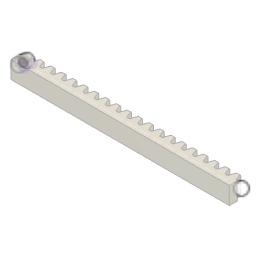
Parametric Rack (Autodesk Fusion 360 design; units mm, degrees)
Autodesk Fusion 360 part; units mm, degrees
sketch "Diameters" plane through (0, 0, 0) normal (0, 1, 0) x (1, 0, 0) in component "Rack"
  line L0 (0, 0) -> (62.8319, 0)
  line L1 (62.8319, 0) -> (62.8319, -4.5)
  line L2 (62.8319, -4.5) -> (0, -4.5)
  line L3 (0, -4.5) -> (0, 0)
  line L4 (0.4803, -2) -> (1.2083, 0)
  line L5 (0.4803, -2) -> (0, -2) construction
  line L6 (1.5708, 0) -> (1.5708, -2.1974) construction
  line L7 (1.2083, 0) -> (1.5708, 0)
  line L8 (2.6613, -2) -> (3.1416, -2) construction
  line L9 (2.6613, -2) -> (1.9333, 0)
  line L10 (1.9333, 0) -> (1.5708, 0)
  line L11 (0, -1) -> (3.1416, -1) construction
  arc A0 (0.1984, -2.1974) -> (0.4803, -2) centre (0.1984, -1.8974) ccw
  line L12 (0.1984, -2.1974) -> (0, -2.1974)
  arc A1 (2.6613, -2) -> (2.9432, -2.1974) centre (2.9432, -1.8974) ccw
  line L13 (2.9432, -2.1974) -> (3.1416, -2.1974)
  line L14 (3.1416, -2.1974) -> (3.1416, 0)
  point P0 (0.8443, -1)
  point P1 (2.2973, -1)
  dimension "d345" = 62.8319
  dimension "d348" = 3.1416
  dimension "d350" = 20
  dimension "d351" = 1.453
  dimension "d352" = 1
  dimension "d353" = 1
  dimension "d354" = 0.3
  dimension "d362" = 4.5
  constraint horizontal L0
  constraint vertical L1
  constraint horizontal L2
  constraint vertical L3
  constraint horizontal L5
  constraint perpendicular L6 L7
  constraint symmetric L4.start L6 L8.start
  constraint symmetric L4.end L6 L9.end
  constraint symmetric L5.end L6 L8.end
  constraint symmetric L7.end L6 L10.end
  constraint perpendicular L6 L11
  constraint coincident L4 P0
  constraint coincident L11 P0
  constraint coincident L11 P1
  constraint coincident L9 P1
  constraint tangent L4 A0
  constraint tangent A0 L12
  constraint vertical L5.end L12.end
  constraint horizontal L12
  constraint horizontal L6.end L12.end
  constraint symmetric L6 A0.start A1.end
  constraint symmetric L6 A0 A1
  constraint symmetric L6 L12.end L13.end
  constraint vertical L5.end L11.start
  constraint vertical L8.end L11.end
  constraint coincident L0 L6.start
  constraint coincident L3 L12.end
  constraint coincident L0.start L3.end
  constraint coincident L0 L14.end
  constraint vertical L14
  measures "d345" distance of L0.start L0.end
  measures "d348" distance of L5.end L8.end
  measures "d350" angle of L4 L6
  measures "d351" distance of P0 P1
  measures "d352" distance of L7 L11
  measures "d353" distance of L5 L11
  measures "d354" radius of A0
  measures "d362" distance of L0.start L2.end
sketch "References" plane through (0, 0, 0) normal (0, 1, 0) x (1, 0, 0) in component "Rack"
  line L0 (1.5708, 0) -> (1.5708, -2.1974) construction
  line L1 (0, -1) -> (62.8319, -1) construction
  line L2 (0, 0) -> (0, -2.1974) construction
  point P0 (0, -1)
  dimension "d364" = 62.8319
  constraint coincident P0 L1.start
  constraint perpendicular L0 L1
  constraint parallel L0 L2
  constraint coincident P0 L2
  constraint horizontal L0.start L2.start
  measures "d364" distance of P0 L1.end
extrude "Create Block" add sketch "Diameters" along normal mid plane 5 in component "Rack"
chamfer "Chamfer1" distance 0.35 angle 45 2 edges at (31.4159, 2.5, 0) (31.4159, -2.5, 0) in component "Rack"
extrude "Create tooth" cut sketch "Diameters" along normal through all and the other way through all contours L0 L3 L4 A0 L12 | L0 L9 A1 L13 L14 in component "Rack"
pattern_linear "R-Pattern1" count 20 spacing 3.1416 along (1, 0, 0) of "Create tooth" in component "Rack"
component "Rack" placed x (1, 0, 0) y (0, 1, 0) z (0, 0, 1) at (0, 0, 0)
equation "RACK_MODULE = 1"
equation "RACK_PRESSURE_ANGLE = 20 deg"
equation "RACK_TEETH = 20"
equation "RACK_THICKNESS = 5 mm"
equation "RACK_FILLET_RADIUS = 0.30 mm * RACK_MODULE"
equation "d222 = RACK_THICKNESS / 2"
equation "RACK_TOOTH_SCALE = 0.925"
equation "RACK_TIP_CHAMFER = 0.35 mm"
equation "d345 = PI mm * RACK_MODULE * RACK_TEETH"
equation "d348 = RACK_MODULE * PI mm"
equation "d350 = RACK_PRESSURE_ANGLE"
equation "d351 = RACK_TOOTH_SCALE * ( RACK_MODULE * PI mm ) / 2"
equation "d352 = 1.0 mm * RACK_MODULE"
equation "d353 = 1.0 mm * RACK_MODULE"
equation "d354 = RACK_FILLET_RADIUS"
equation "d357 = RACK_TIP_CHAMFER"
equation "d358 = RACK_TEETH"
equation "d360 = -PI mm * RACK_MODULE"
equation "d362 = RACK_HEIGHT"
equation "RACK_HEIGHT = 2.25 mm * RACK_MODULE * 2"
equation "d364 = PI mm * RACK_MODULE * RACK_TEETH"
named bodies: "Rack"
